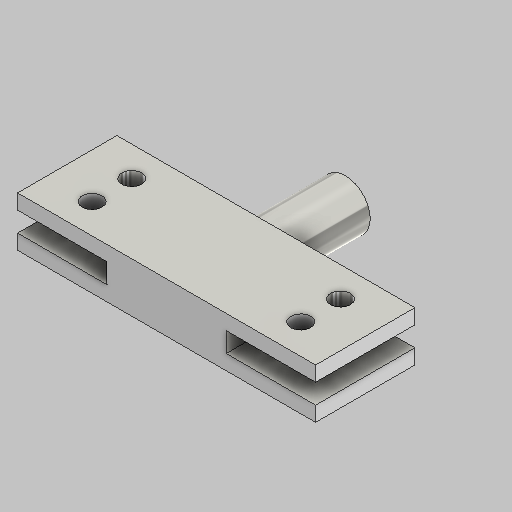
# Autodesk Inventor part: Junta
Saved by Autodesk Inventor 2025.2 (Build 292293000, 293)
## iProperties
Created: 2024-04-26
Part Number: Junta
Material: Genérico
Document SubType Name: Modeling
Designer: phmca
Density: 1 g/cm^3
Appearance: Padrão
Author: phmca
Autodesk Inventor part; units mm, degrees
ref_plane "YZ Plane" through (0, 0, 0) normal (1, 0, 0) x (0, 1, 0)
ref_plane "XZ Plane" through (0, 0, 0) normal (0, 1, 0) x (-1, 0, 0)
ref_plane "XY Plane" through (0, 0, 0) normal (0, 0, 1) x (1, 0, 0)
sketch "Esboço1" plane through (0, 0, 0) normal (0, 0, 1) x (1, 0, 0)
  circle A0 centre (0, 0) radius 12.5
  arc A1 (0, 12.5) -> (0, 12.5) centre (0, 0) ccw
  line L0 (0, 12.5) -> (75, 12.5)
  line L1 (75, 12.5) -> (75, 5)
  line L2 (0, -12.5) -> (75, -12.5)
  line L3 (75, -12.5) -> (75, -5)
  line L4 (75, 5) -> (30, 5)
  line L5 (30, -5) -> (75, -5)
  line L6 (75, -5) -> (75, 5) construction
  line L7 (75, 0) -> (28.253, 0) construction
  line L8 (0, 0) -> (-5.8343, 0) construction
  arc A2 (11.9242, 3.75) -> (0, 12.5) centre (0, 0) ccw construction
  arc A3 (0, -12.5) -> (11.9242, -3.75) centre (0, 0) ccw construction
  arc A4 (11.9242, -3.75) -> (11.9242, 3.75) centre (0, 0) ccw construction
  line L9 (0, 0) -> (0, 31.0423) construction
  line L10 (0, 12.5) -> (-75, 12.5)
  line L11 (0, -12.5) -> (-75, -12.5)
  line L12 (-75, -12.5) -> (-75, -5)
  line L13 (-75, 5) -> (-30, 5)
  line L14 (-30, -5) -> (-75, -5)
  line L15 (-75, 5) -> (-75, 12.5)
  arc A5 (0, 12.5) -> (-11.9242, 3.75) centre (0, 0) ccw construction
  arc A6 (-11.9242, 3.75) -> (-11.9242, -3.75) centre (0, 0) ccw construction
  arc A7 (-11.9242, -3.75) -> (0, -12.5) centre (0, 0) ccw construction
  arc A8 (0, -12.5) -> (0, -12.5) centre (0, 0) ccw
  line L16 (30, -5) -> (30, 5)
  line L17 (-30, -5) -> (-30, 5)
  arc A9 (0, 12.5) -> (0, 12.5) centre (0, 22.5) ccw
  arc A10 (0, -12.5) -> (0, -12.5) centre (0, -22.5) ccw
  arc A11 (0, -12.5) -> (0, -12.5) centre (0, -22.5) ccw
  arc A12 (0, 12.5) -> (0, 12.5) centre (0, 22.5) ccw
  line L18 (-30, 0) -> (30, 0)
  line L19 (0, 0) -> (0, 17) construction
  dimension "d0" = 25
  dimension "d1" = 25
  dimension "d6" = 10
  dimension "d7" = 7.5
  dimension "d8" = 7.5
  dimension "d10" = 10
  dimension "d13" = 150
  dimension "d45" = 60
  constraints: 40 end point, 29 point on circle, 13 centre point, 8 symmetric about line, 8 tangent, 6 collinear, 6 perpendicular, 6 point on line, 4 horizontal, 4 midpoint, 3 equal radius, 3 vertical, 2 coincident, 1 parallel
  measures "d0" diameter of A0
  measures "d1" diameter of A1
  measures "d6" distance between parallel lines of L5 L4
  measures "d7" distance of L0.end L1.end
  measures "d8" distance of L2.end L3.end
  measures "d10" radius of A9
  measures "d13" distance between parallel lines of L1 L15
  measures "d45" distance between parallel lines of L16 L17
extrude "Extrusão1" add sketch "Esboço1" along normal blind 50 contours L18 A0 | L18 L16 L5 L3 L2 A0 | A0 L0 L1 L4 L16 L18 | A0 L18 | A0 L18 L17 L13 L15 L10 | L11 L12 L14 L17 L18 A0
extrude "Extrusão2" add sketch "Esboço1" against normal blind 40 contours L18 A0 | A0 L18
sketch "Esboço2" plane through (0, 12.5, 0) normal (0, 1, 0) x (1, 0, 0)
  circle A0 centre (52.5, -15) radius 5
  circle A1 centre (-52.5, -15) radius 5
  line L0 (75, 0) -> (75, -50) projected
  line L1 (-75, 0) -> (-75, -50) projected
  circle A2 centre (-52.5, -35) radius 5
  circle A3 centre (52.5, -35) radius 5
  line L2 (0, 0) -> (-75, 0) projected
  line L3 (-52.5, -35) -> (-52.5, -15) construction
  line L4 (75, 0) -> (0, 0) projected
  line L5 (52.5, -35) -> (52.5, -15) construction
  dimension "d17" = 10
  dimension "d18" = 10
  dimension "d22" = 150
  dimension "d23" = 22.5
  dimension "d29" = 22.5
  dimension "d38" = 10
  dimension "d40" = 20
  dimension "d41" = 10
  dimension "d44" = 20
  dimension "d63" = 15
  dimension "d64" = 15
  constraints: 4 centre point, 4 end point, 2 vertical
  measures "d17" diameter of A0
  measures "d18" diameter of A1
  measures "d22" distance between parallel lines of L0 L1
  measures "d23" distance from line of L1 L3.end
  measures "d29" distance from line of L0 L5.end
  measures "d38" diameter of A2
  measures "d40" distance of L3.end L3.start
  measures "d41" diameter of A3
  measures "d44" distance of L5.start L5.end
  measures "d63" distance from line of L2 L3.end
  measures "d64" distance from line of L4 L5.end
extrude "Extrusão3" cut sketch "Esboço2" against normal up to surface (25 mm away)
sketch "Esboço4" plane through (-75, -12.5, 50) normal (0, -1, 0) x (1, 0, 0)
  circle A0 centre (47.5, -25) radius 2.5
  circle A1 centre (102.5, -25) radius 2.5
  line L0 (47.5, -25) -> (102.5, -25)
  line L1 (75, -25) -> (75, -15.8254)
  line L2 (150, 0) -> (0, 0) projected
  line L3 (75, 0) -> (75, 11.0535)
  line L4 (0, -50) -> (0, 0) projected
  line L5 (0, -25) -> (-11.4925, -25)
  point P0 (75, -50)
  dimension "d53" = 5
  dimension "d54" = 5
  dimension "d55" = 55
  constraints: 8 end point, 3 midpoint, 2 centre point, 2 collinear, 2 horizontal, 2 vertical
  measures "d53" diameter of A0
  measures "d54" diameter of A1
  measures "d55" distance of L0.start L0.end
hole "Furo2" at (-27.5, -12.5, 25) at (27.5, -12.5, 25) direction (0, 1, 0) diameter 4.134 depth 5 tip angle 118 thread size "M5x0.8" class "6H" standard "ISO Metric profile"
equation "\"d8\" = d7"
equation "\"d29\" = d23"
equation "\"d38\" = d18"
equation "\"d41\" = d17"
